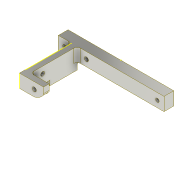
# Autodesk Inventor part: middleMountBracket
Saved by Autodesk Inventor 2020 (Build 240168000, 168)
## iProperties
Created: 2019-12-23
Part Number: middleMountBracket
Material: Silver
Document SubType Name: Modeling
Designer: FTC8863
Density: 10.49 g/cm^3
Appearance: Silver
Mass: 179.682 g
Surface Area: 80.074 cm^2
Volume: 17.1289 cm^3
Author: FTC8863
Autodesk Inventor part; units mm, degrees
ref_plane "YZ Plane" through (0, 0, 0) normal (1, 0, 0) x (0, 1, 0)
ref_plane "XZ Plane" through (0, 0, 0) normal (0, 1, 0) x (-1, 0, 0)
ref_plane "XY Plane" through (0, 0, 0) normal (0, 0, 1) x (1, 0, 0)
sketch "Sketch1" plane through (0, 0, 0) normal (0, 0, 1) x (1, 0, 0)
  line L0 (-50.8, 6.35) -> (-50.8, -6.35)
  line L1 (-50.8, -6.35) -> (50.8, -6.35)
  line L2 (50.8, -6.35) -> (50.8, 6.35)
  line L3 (50.8, 6.35) -> (-50.8, 6.35)
  point P0 (0, 0)
  dimension "d0" = 101.6
  dimension "d1" = 12.7
  dimension "d2" = 50.8
  dimension "d3" = 6.35
  constraints: 8 end point, 3 perpendicular, 1 vertical
  measures "d0" distance of L2.end L0.start
  measures "d1" distance of L1.end L2.end
  measures "d2" distance from line of point (0, 0) L2
  measures "d3" distance from line of point (0, 0) L3
extrude "Extrusion1" add sketch "Sketch1" along normal blind 9.398
sketch "Sketch2" plane through (0, 0, 9.398) normal (0, 0, 1) x (1, 0, 0)
  line L0 (-38.1, 6.35) -> (-38.1, -6.35)
  line L1 (-50.8, -6.35) -> (50.8, -6.35) projected
  line L2 (-50.8, 6.35) -> (-50.8, -6.35) projected
  line L3 (-38.1, 6.35) -> (-32.6898, 6.35)
  line L4 (50.8, 6.35) -> (-50.8, 6.35) projected
  line L5 (-38.1, 6.35) -> (-32.6898, 6.35) construction
  line L6 (-32.6898, 6.35) -> (-32.6898, -6.35)
  line L7 (-38.1, -6.35) -> (-32.6898, -6.35)
  point P0 (0, 0)
  point P1 (-38.1, -6.35)
  dimension "d6" = 12.7
  dimension "d8" = 5.4102
  dimension "d9" = 0
  constraints: 10 end point, 2 collinear, 2 perpendicular, 1 horizontal, 1 point on line, 1 vertical
  measures "d6" distance between parallel lines of L2 L0
  measures "d8" distance of L0.start L3.end
  measures "d9" distance between parallel lines of L5 L3
extrude "Extrusion2" add sketch "Sketch2" along normal blind 50.0888 contours L3 L6 L1 L0
sketch "Sketch3" plane through (-32.6898, -6.35, 9.398) normal (1, 0, 0) x (0, 0, -1)
  line L0 (0, 12.7) -> (-50.0888, 12.7) projected
  line L1 (0, 0) -> (-50.0888, 0) projected
  line L2 (-50.0888, 12.7) -> (-50.0888, 0) projected
  line L3 (-50.0888, 12.7) -> (-50.0888, 0)
  line L4 (-50.0888, 0) -> (-44.6786, 0)
  line L5 (-44.6786, 0) -> (-44.6786, 12.7)
  line L6 (-44.6786, 12.7) -> (-50.0888, 12.7)
  point P0 (9.398, 6.35)
  dimension "d14" = 5.4102
  constraints: 8 end point, 2 collinear, 2 point on line, 1 perpendicular
  measures "d14" distance of L1.end L4.end
extrude "Extrusion3" add sketch "Sketch3" along normal blind 17.8308
sketch "Sketch4" plane through (-50.8, 6.35, 0) normal (0, 1, 0) x (1, 0, 0)
  point P0 (50.8, 0)
sketch "Sketch5" plane through (0, 0, 9.398) normal (0, 0, 1) x (1, 0, 0)
  circle A0 centre (-44.7923, 0) radius 1.6993
  line L0 (-50.8, -6.35) -> (-38.1, -6.35) projected
  point P0 (0, 0)
  dimension "d17" = 3.3985
  dimension "d18" = 6.35
  constraints: 1 centre point
  measures "d17" diameter of A0
  measures "d18" distance from line of L0 A0.centre
extrude "Extrusion4" cut sketch "Sketch5" against normal blind 17.8308
sketch "Sketch6" plane through (0, 0, 9.398) normal (0, 0, 1) x (1, 0, 0)
  circle A0 centre (44.45, 0) radius 1.6993
  line L0 (50.8, -6.35) -> (50.8, 6.35) projected
  point P0 (0, 0)
  dimension "d21" = 3.3985
  dimension "d22" = 6.35
  constraints: 1 centre point
  measures "d21" diameter of A0
  measures "d22" distance from line of L0 A0.centre
extrude "Extrusion5" cut sketch "Sketch6" against normal blind 17.8308
sketch "Sketch7" plane through (0, 0, 59.4868) normal (0, 0, 1) x (1, 0, 0)
  circle A0 centre (-23.7744, 0) radius 1.9685
  line L0 (-14.859, 6.35) -> (-14.859, -6.35) projected
  point P0 (0, 0)
  dimension "d25" = 3.937
  dimension "d26" = 8.9154
  constraints: 1 centre point
  measures "d25" diameter of A0
  measures "d26" distance from line of L0 A0.centre
extrude "Extrusion6" cut sketch "Sketch7" against normal blind 76.2
sketch "Sketch8" plane through (-50.8, -6.35, 0) normal (0, -1, 0) x (1, 0, 0)
  line L0 (18.1102, 54.0766) -> (35.941, 54.0766) projected
  line L1 (18.1102, 54.0766) -> (14.954, 54.0766)
  line L2 (14.954, 54.0766) -> (14.954, 9.398)
  line L3 (18.1102, 9.398) -> (18.1102, 54.0766) projected
  line L4 (14.954, 9.398) -> (18.1102, 9.398)
  line L5 (18.1102, 9.398) -> (18.1102, 54.0766)
  point P0 (50.8, 0)
  constraints: 8 end point, 2 perpendicular, 1 horizontal, 1 parallel
extrude "Extrusion7" add sketch "Sketch8" along normal blind 19.812
sketch "Sketch9" plane through (-32.6898, 6.35, 54.0766) normal (1, 0, 0) x (0, 0, -1)
  point P0 (54.0766, -6.35)
sketch "Sketch10" plane through (-32.6898, 6.35, 54.0766) normal (1, 0, 0) x (0, 0, -1)
  line L0 (0, -32.512) -> (44.6786, -32.512) projected
  line L1 (4.5681, -32.512) -> (4.5681, -15.2301)
  line L2 (4.5681, -15.2301) -> (18.5381, -15.2301)
  line L3 (18.5381, -15.2301) -> (18.5381, -32.512)
  line L4 (4.5681, -32.512) -> (18.5381, -32.512)
  point P0 (54.0766, -6.35)
  dimension "d31" = 13.97
  constraints: 8 end point, 4 perpendicular, 2 point on line
  measures "d31" distance of L1.end L2.end
extrude "Extrusion8" cut sketch "Sketch10" against normal blind 19.812
sketch "Sketch13" plane through (0, 0, 0) normal (0, 0, -1) x (-1, 0, 0)
  point P0 (0, 0)
sketch "Sketch15" plane through (0, 0, 0) normal (0, 0, -1) x (-1, 0, 0)
  circle A0 centre (23.7744, 0) radius 1.9685 projected
  circle A1 centre (23.7744, 0) radius 4.6609 construction
  line L0 (19.1135, 0) -> (21.4439, 4.0365)
  line L1 (21.4439, 4.0365) -> (26.1048, 4.0365)
  line L2 (26.1048, 4.0365) -> (28.4353, 0)
  line L3 (28.4353, 0) -> (26.1049, -4.0365)
  line L4 (26.1049, -4.0365) -> (21.444, -4.0365)
  line L5 (21.444, -4.0365) -> (19.1135, 0)
  point P0 (0, 0)
  dimension "d83" = 9.3218
  constraints: 12 end point, 3 coincident, 1 horizontal alignment, 15 other
extrude "Extrusion11" cut sketch "Sketch15" against normal blind 4.826 contours A0 | L0 L1 L2 L3 L4 L5
sketch "Sketch17" plane through (-38.1, -6.35, 9.398) normal (-1, 0, 0) x (0, 0, 1)
  line L0 (40.1105, -2.5301) -> (26.1405, -2.5301) projected
  line L1 (33.1255, -2.5301) -> (33.1255, 12.7)
  line L2 (0, 12.7) -> (44.6786, 12.7) projected
  line L3 (50.0888, 12.7) -> (50.0888, 0) projected
  line L4 (50.0888, 6.35) -> (0, 6.35)
  line L5 (0, 8.0493) -> (0, 4.6507) projected
  point P0 (-9.398, 6.35)
  constraints: 4 end point, 3 midpoint, 1 point on line, 1 vertical
sketch "Sketch19" plane through (-38.1, -6.35, 9.398) normal (-1, 0, 0) x (0, 0, 1)
  point P0 (-9.398, 6.35)
  point P1 (33.1582, 6.3688)
hole "Hole3" at (-38.1, 0.0188, 42.5562) direction (1, 0, 0) diameter 3.81 end through all
fillet "Fillet1" radius 3.175 1 edges at (-35.846, -6.35, 31.7373)
fillet "Fillet2" radius 3.175 1 edges at (-35.3949, -6.35, 54.0766)
fillet "Fillet3" radius 3.175 1 edges at (-35.3949, -6.35, 9.398)
fillet "Fillet4" radius 3.175 1 edges at (-38.1, 0, 9.398)
fillet "Fillet5" radius 3.175 1 edges at (-32.6898, 0, 54.0766)
fillet "Fillet6" radius 3.175 1 edges at (-32.6898, 0, 9.398)
sketch "Sketch20" plane through (-32.6898, -26.162, 49.5085) normal (1, 0, 0) x (0, 0, -1)
  line L0 (0, 17.2819) -> (13.97, 17.2819) projected
  line L1 (0, 17.2819) -> (-7.9375, 17.2819)
  line L2 (-7.9375, 17.2819) -> (-9.525, -14.2875)
  line L3 (-9.525, -14.2875) -> (9.525, -12.7)
  line L4 (9.525, -12.7) -> (0, 17.2819)
  point P0 (49.5085, 26.162)
  constraints: 8 end point, 1 horizontal
extrude "Extrusion12" cut sketch "Sketch20" against normal blind 25.4
sketch "Sketch21" plane through (-32.6898, -26.162, 35.5385) normal (1, 0, 0) x (0, 0, -1)
  line L0 (0, 0) -> (0, 16.7735) projected
  line L1 (0, 12.7) -> (26.1405, 12.7)
  line L2 (26.1405, 16.637) -> (26.1405, 0) projected
  line L3 (26.1405, 12.7) -> (39.6875, -1.5875)
  line L4 (39.6875, -1.5875) -> (35.1397, -17.3529)
  line L5 (35.1397, -17.3529) -> (19.05, -19.05)
  line L6 (19.05, -19.05) -> (9.525, -9.0044)
  line L7 (9.525, -9.0044) -> (7.9375, -26.9875)
  line L8 (7.9375, -26.9875) -> (-2.7297, -30.1625)
  line L9 (-2.7297, -30.1625) -> (-7.3449, -19.05)
  line L10 (-7.3449, -19.05) -> (-5.0373, -4.7625)
  line L11 (-5.0373, -4.7625) -> (0, 12.7)
  point P0 (35.5385, 26.162)
  constraints: 20 end point, 2 parallel, 2 point on line, 1 horizontal
extrude "Extrusion13" cut sketch "Sketch21" against normal blind 25.4
sketch "Sketch22" plane through (0, 0, 59.4868) normal (0, 0, 1) x (1, 0, 0)
  line L0 (-29.5148, -6.35) -> (50.8, -6.35) projected
  line L1 (-14.859, -6.35) -> (-14.859, 6.35) projected
  arc A0 (-20.6375, -6.35) -> (-14.859, 0) centre (-49.851, 26.0385) ccw
  line L2 (-20.6375, -6.35) -> (-17.4625, -11.1125)
  line L3 (-17.4625, -11.1125) -> (-11.1125, -4.7625)
  line L4 (-11.1125, -4.7625) -> (-14.859, 0)
  point P0 (0, 0)
  point P1 (-12.7, -6.35)
  constraints: 6 end point, 2 point on circle, 1 centre point, 1 midpoint, 1 point on line
extrude "Extrusion14" cut sketch "Sketch22" against normal blind 25.4 contours A0 L1 L0 | L1 L4 L3 L0
sketch "Sketch23" plane through (0, 0, 59.4868) normal (0, 0, 1) x (1, 0, 0)
  line L0 (-38.1, -6.35) -> (-20.6375, -6.35) projected
  line L1 (-23.8125, -6.35) -> (-17.4625, -3.175)
  arc A0 (-20.6375, -6.35) -> (-14.859, 0) centre (-49.851, 26.0385) ccw projected
  line L2 (-15.875, -9.525) -> (-19.05, -12.7)
  line L3 (-19.05, -12.7) -> (-23.8125, -9.525)
  line L4 (-23.8125, -9.525) -> (-20.6375, -7.9375)
  line L5 (-20.6375, -7.9375) -> (-23.8125, -6.35)
  line L6 (-17.4625, -3.175) -> (-15.875, -9.525)
  point P0 (0, 0)
  constraints: 12 end point, 3 point on line, 2 point on circle
extrude "Extrusion15" cut sketch "Sketch23" along normal blind 25.4 and the other way blind 12.7
sketch "Sketch24" plane through (0, 0, 59.4868) normal (0, 0, 1) x (1, 0, 0)
  line L0 (-29.5148, -6.35) -> (-23.8125, -6.35) projected
  arc A0 (-17.4625, -3.175) -> (-14.859, 0) centre (-49.851, 26.0385) ccw projected
  line L1 (-17.4625, -3.175) -> (-23.8125, -6.35) projected
  arc A1 (-23.8125, -6.35) -> (-14.859, 0) centre (-26.4391, 6.8408) ccw
  line L2 (-14.859, 0) -> (-14.859, 6.35) projected
  line L3 (-23.8125, -6.35) -> (-14.859, 0)
  point P0 (0, 0)
  constraints: 3 point on circle, 2 end point, 1 centre point
extrude "Extrusion16" add sketch "Sketch24" against normal blind 5.4102
fillet "Fillet7" radius 3.175 2 edges at (-14.859, 0, 56.7817) (-23.8125, -6.35, 56.7817)
body "Solid1"
